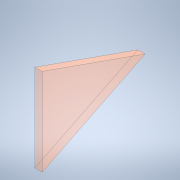
# Autodesk Inventor part: HPSFlagPurple-ver1-1111-2021
Saved by Autodesk Inventor 2021 (Build 250183000, 183)
## iProperties
Created: 2021-03-04
Part Number: HPSFlagPurple-ver1-1111-2021
Material: Generic
Document SubType Name: Modeling
Designer: CMurray
Density: 1 g/cm^3
Appearance: Polycarbonate - Clear
Author: CMurray
Autodesk Inventor part; units mm, degrees
ref_plane "YZ Plane" through (0, 0, 0) normal (1, 0, 0) x (0, 1, 0)
ref_plane "XZ Plane" through (0, 0, 0) normal (0, 1, 0) x (-1, 0, 0)
ref_plane "XY Plane" through (0, 0, 0) normal (0, 0, 1) x (1, 0, 0)
sketch "Sketch2" plane through (0, 0, 0) normal (1, 0, 0) x (0, 1, 0)
  line L0 (0, 0) -> (304.8, 0)
  line L1 (304.8, 0) -> (177.8, -359.2102)
  line L2 (177.8, -359.2102) -> (0, 0)
  dimension "d1" = 304.8
  dimension "d2" = 381
  constraints: 6 end point, 1 horizontal
  measures "d1" distance of L0.start L0.end
  measures "d2" distance of L0.end L1.end
extrude "Extrusion1" add sketch "Sketch2" along normal blind 25.4
body "Solid1"
